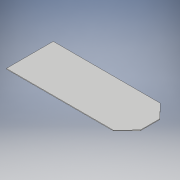
# Autodesk Inventor part: 140x55mm-PCB
Saved by Autodesk Inventor 2018 (Build 220112000, 112)
## iProperties
Created: 2018-04-06
Part Number: 140x55mm-PCB
Material: Generic
Document SubType Name: Modeling
Designer: bbramman
Density: 1 g/cm^3
Appearance: Default
Author: bbramman
Autodesk Inventor part; units mm, degrees
ref_plane "YZ Plane" through (0, 0, 0) normal (1, 0, 0) x (0, 1, 0)
ref_plane "XZ Plane" through (0, 0, 0) normal (0, 1, 0) x (-1, 0, 0)
ref_plane "XY Plane" through (0, 0, 0) normal (0, 0, 1) x (1, 0, 0)
sketch "Sketch1" plane through (0, 0, 0) normal (0, 1, 0) x (-1, 0, 0)
  line L0 (-60.5593, 27.4889) -> (62.6411, -28.4339) construction
  line L1 (62.6424, 27.1286) -> (-64.3576, -27.8714) construction
  line L2 (-77.4954, -16.5) -> (-44.4954, -16.5) construction
  line L3 (-63.5, 27.7812) -> (63.5, 27.7812)
  line L4 (63.5, 27.7812) -> (63.5, -27.7812)
  line L5 (63.5, -27.7812) -> (-63.5, -27.7812)
  line L6 (-63.5, 27.7812) -> (63.5, -27.7812) construction
  line L7 (63.5, 27.7812) -> (-63.5, -27.7812) construction
  line L8 (-63.5, 11.5094) -> (63.5, 11.5094)
  line L9 (63.5, 11.5094) -> (63.5, -11.5094)
  line L10 (63.5, -11.5094) -> (-63.5, -11.5094)
  line L11 (-63.5, 11.5094) -> (63.5, -11.5094) construction
  line L12 (63.5, 11.5094) -> (-63.5, -11.5094) construction
  line L13 (-79.375, 11.5094) -> (-79.375, -11.5094)
  line L14 (-63.5, 27.7812) -> (-79.375, 11.5094)
  line L15 (-79.375, -11.5094) -> (-63.5, -27.7812)
  point P0 (0, 0)
  dimension "d1" = 55.5625
  dimension "d6" = 127
  dimension "d7" = 55.5625
  dimension "d8" = 127
  dimension "d9" = 23.0188
  constraints: 32 end point, 4 midpoint, 3 horizontal, 2 parallel, 2 perpendicular, 2 point on line
  measures "d1" distance of L1.start L0.end
  measures "d6" distance of L4.end L5.end
  measures "d7" distance of L3.end L4.end
  measures "d8" distance of L9.end L10.end
  measures "d9" distance of L8.end L9.end
extrude "Extrusion1" add sketch "Sketch1" along normal mid plane 0.7874
body "Solid1"
